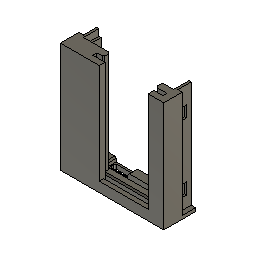
POWERDIAG_OBI_CASE_1 (Autodesk Fusion 360 design; units mm, degrees)
part number: 2026-08-31-19-42-01-999
Autodesk Fusion 360 part; units mm, degrees
note: some values were not read from the file. Set by a fixed rule: which sketch regions a step uses.
sketch "Sketch1" plane through (0, 0, 0) normal (0, 0, 1) x (1, 0, 0)
  line L0 (0, 0) -> (46.5, 0)
  line L1 (46.5, 0) -> (46.5, 14.3)
  line L2 (46.5, 14.3) -> (0, 14.3)
  line L3 (0, 14.3) -> (0, 0)
  line L4 (0, 2.6) -> (46.5, 2.6)
  line L5 (3, 14.3) -> (3, 0)
  line L6 (43.5, 14.3) -> (43.5, 0)
  line L7 (0, 4.4) -> (46.5, 4.4)
  line L8 (0, 7.4) -> (46.5, 7.4)
  line L9 (10.8, 10.6) -> (19.8, 10.6)
  line L10 (19.8, 10.6) -> (19.8, 14.3)
  line L11 (19.8, 14.3) -> (10.8, 14.3)
  line L12 (10.8, 14.3) -> (10.8, 10.6)
  line L13 (4, 10.6) -> (4, 9)
  line L14 (4, 9) -> (3, 9)
  line L15 (3, 9) -> (3, 11)
  line L16 (42.5, 10.6) -> (42.5, 9)
  line L17 (42.5, 9) -> (43.5, 9)
  line L18 (43.5, 9) -> (43.5, 11)
  line L19 (6.8, 14.3) -> (23.8, 14.3)
  line L20 (43.5, 10.6) -> (3, 10.6)
  line L21 (11.2, 13.45) -> (19.4, 13.45)
  line L22 (19.4, 13.45) -> (19.4, 10.95)
  line L23 (19.4, 10.95) -> (11.2, 10.95)
  line L24 (11.2, 10.95) -> (11.2, 13.45)
  line L25 (12, 4.4) -> (12, 2.6)
  line L26 (15, 7.4) -> (15, 4.4)
  line L27 (38.5, 7.4) -> (38.5, 4.4)
  line L28 (17.5, 2.6) -> (17.5, 0)
  line L29 (39.5, 2.6) -> (39.5, 0)
  line L30 (4, 10.6) -> (4, 14.3)
  line L31 (42.5, 10.6) -> (42.5, 14.3)
  dimension "d3" = 2.6
  dimension "d4" = 3
  dimension "d5" = 3
  dimension "d7" = 1.8
  dimension "d8" = 3
  dimension "d9" = 3.2
  dimension "d10" = 3.7
  dimension "d11" = 9
  dimension "d12" = 7.8
  dimension "d13" = 40.5
  dimension "d23" = 1
  dimension "d24" = 1.6
  dimension "d25" = 1.6
  dimension "d26" = 1
  dimension "d34" = 8.2
  dimension "d35" = 2.5
  dimension "d36" = 0.4
  dimension "d37" = 0.85
  dimension "d42" = 9
  dimension "d43" = 12
  dimension "d44" = 5
  dimension "d45" = 14.5
  dimension "d46" = 4
  constraint horizontal L0
  constraint vertical L1
  constraint horizontal L2
  constraint vertical L3
  constraint coincident L0.start L3.end
  constraint coincident L3 L4.start
  constraint coincident L1 L4.end
  constraint perpendicular L1 L4
  constraint coincident L2 L5.start
  constraint coincident L0 L5.end
  constraint perpendicular L0 L5
  constraint coincident L2 L6.start
  constraint coincident L0 L6.end
  constraint perpendicular L0 L6
  constraint coincident L1 L7.end
  constraint perpendicular L1 L7
  constraint coincident L3 L8.start
  constraint perpendicular L6 L8
  constraint coincident L1 L8.end
  constraint horizontal L9
  constraint vertical L10
  constraint horizontal L11
  constraint vertical L12
  constraint vertical L13
  constraint horizontal L14
  constraint vertical L15
  constraint coincident L5 L15.end
  constraint vertical L16
  constraint horizontal L17
  constraint vertical L18
  constraint coincident L6 L18.end
  constraint horizontal L19
  constraint horizontal L20
  constraint collinear L9 L20
  constraint horizontal L21
  constraint vertical L22
  constraint horizontal L23
  constraint vertical L24
  constraint coincident L7 L25.start
  constraint coincident L4 L25.end
  constraint perpendicular L7 L25
  constraint coincident L8 L26.start
  constraint coincident L7 L26.end
  constraint perpendicular L7 L26
  constraint coincident L8 L27.start
  constraint coincident L7 L27.end
  constraint perpendicular L7 L27
  constraint coincident L4 L28.start
  constraint coincident L0 L28.end
  constraint perpendicular L0 L28
  constraint coincident L4 L29.start
  constraint coincident L0 L29.end
  constraint perpendicular L0 L29
  constraint collinear L11 L19
  constraint collinear L2 L11
  constraint coincident L15 L20.end
  constraint coincident L16.start L20
  constraint coincident L13.start L20
  constraint coincident L2 L30.end
  constraint perpendicular L2 L30
  constraint coincident L2 L31.end
  constraint perpendicular L2 L31
  measures "d3" distance of L0 L4
  measures "d4" distance of L3 L5
  measures "d5" distance of L1 L6
  measures "d7" distance of L4 L7
  measures "d8" distance of L7 L8
  measures "d9" distance of L8 L9
  measures "d10" distance of L9.start L11.end
  measures "d11" distance of L10 L12
  measures "d12" distance of L5 L12
  measures "d13" distance of L5 L6
  measures "d23" distance of L5 L13
  measures "d24" distance of L8 L14
  measures "d25" distance of L8 L17
  measures "d26" distance of L16 L18
  measures "d34" distance of L22 L24
  measures "d35" distance of L21 L23
  measures "d36" distance of L12 L24
  measures "d37" distance of L11 L21
  measures "d42" distance of L5 L25
  measures "d43" distance of L5 L26
  measures "d44" distance of L6 L27
  measures "d45" distance of L5 L28
  measures "d46" distance of L6 L29
extrude "Extrude1" add sketch "Sketch1" against normal blind 2
extrude "Extrude2" add sketch "Sketch1" along normal blind 3 contours L0 L3 L4 L5 | L0 L4 L5 L28 | L3 L4 L5 L7 | L0 L4 L28 L29 | L3 L5 L7 L8 | L0 L4 L6 L29 | L5 L7 L8 L26 | L2 L3 L5 L8 L15 | L0 L1 L4 L6 | L1 L4 L6 L7 | L7 L8 L26 L27 | L6 L7 L8 L27 | L1 L6 L7 L8 | L1 L2 L6 L8 L18
sketch "Sketch2" plane through (0, 0, 3) normal (0, 0, 1) x (-1, 0, 0)
  line L0 (-3, -4.4) -> (-43.5, -4.4)
  line L1 (-43.5, -4.4) -> (-43.5, -2.6)
  line L2 (-43.5, -2.6) -> (-3, -2.6)
  line L3 (-3, -2.6) -> (-3, -4.4)
  line L4 (0, -14.3) -> (0, 0)
  line L5 (0, 0) -> (-46.5, 0)
  line L6 (-46.5, 0) -> (-46.5, -14.3)
  line L7 (-43.5, -14.3) -> (-43.5, -7.4)
  line L8 (-43.5, -7.4) -> (-3, -7.4)
  line L9 (-3, -7.4) -> (-3, -14.3)
  line L10 (-15, -7.4) -> (-15, -4.4)
  line L11 (-3, -14.3) -> (-3, 0)
  line L12 (-38.5, -7.4) -> (-38.5, -4.4)
  line L13 (-43.5, -14.3) -> (-43.5, 0)
  line L14 (-12, -4.4) -> (-12, -2.6)
  line L15 (-38.5, -7.4) -> (-38.5, -4.4)
  line L16 (-15, -7.4) -> (-15, -4.4)
  line L17 (-17.5, -2.6) -> (-17.5, 0)
  line L18 (-39.5, -2.6) -> (-39.5, 0)
  line L19 (-3, -14.3) -> (0, -14.3)
  line L20 (-46.5, -14.3) -> (-43.5, -14.3)
  dimension "d18" = 12
  dimension "d19" = 5
  constraint coincident L8 L10.start
  constraint coincident L0 L10.end
  constraint perpendicular L0 L10
  constraint coincident L8 L12.start
  constraint coincident L0 L12.end
  constraint perpendicular L0 L12
  measures "d18" distance of L10 L11
  measures "d19" distance of L12 L13
extrude "Extrude3" add sketch "Sketch2" along normal blind 45 contours L0 L8 L10 L11 L16 | L0 L2 L3 L11 L14 | L3 L4 L5 L9 L11 L19 | L2 L5 L11 L17 | L0 L8 L12 L13 L15 | L1 L5 L6 L7 L13 L20 | L2 L5 L13 L18
extrude "Extrude4" add sketch "Sketch1" along normal blind 45 contours L5 L13 L14 L15 L20 | L2 L5 L15 L20 L30 | L6 L16 L17 L18 L20 | L2 L6 L18 L20 L31
chamfer "Chamfer1" distance 0.6 angle 45 8 edges at (4, 9, 22.5) (15, 7.4, 25.5) (15, 4.4, 25.5) (42.5, 9, 22.5) (38.5, 7.4, 25.5) (38.5, 4.4, 25.5) (28.5, 2.6, 3) (26.75, 4.4, 3)
extrude "Extrude5" add sketch "Sketch1" along normal blind 2 contours L2 L5 L15 L20 L30 | L2 L12 L19 L20 L30 | L2 L6 L18 L20 L31 | L2 L10 L19 L20 L31
fillet "Fillet1" radius 0.8 4 edges at (11.2, 10.95, -1) (19.4, 10.95, -1) (19.4, 13.45, -1) (11.2, 13.45, -1)
extrude "Extrude6" cut sketch "Sketch1" against normal blind 0.5 contours L5 L6 L8 L9 L13 L14 L16 L17 L20
chamfer "Chamfer2" distance 0.6 angle 45 2 edges at (10.8, 12.45, 2) (19.8, 12.45, 2)
sketch "Sketch3" plane through (0, 0, 0) normal (-1, 0, 0) x (0, -1, 0)
  line L0 (-14.3, 48) -> (-14.3, -2)
  line L1 (-14.3, -2) -> (0, -2)
  line L2 (0, -2) -> (0, 48)
  line L3 (0, 48) -> (-14.3, 48)
  line L4 (-8.3, 0) -> (-14.3, 0)
  line L5 (-14.3, 0) -> (-14.3, 48)
  line L6 (-14.3, 48) -> (-8.3, 48)
  line L7 (-8.3, 48) -> (-8.3, 0)
  line L8 (-14.3, 0) -> (0, 0)
  dimension "d52" = 6
  constraint horizontal L4
  constraint vertical L5
  constraint horizontal L6
  constraint vertical L7
  constraint coincident L0.start L3.end
  constraint collinear L4 L8
  measures "d52" distance of L5 L7
extrude "Extrude7" cut sketch "Sketch3" against normal blind 2 contours L0 L3 L4 L5 L6 L7 L8
sketch "Sketch4" plane through (46.5, 0, 0) normal (1, 0, 0) x (0, 1, 0)
  line L0 (0, 48) -> (0, -2)
  line L1 (0, -2) -> (14.3, -2)
  line L2 (14.3, -2) -> (14.3, 48)
  line L3 (14.3, 48) -> (0, 48)
ref_plane "WorkPlane1" through (23.25, 7.15, 23) normal (-1, 0, 0) x (0, 1, 0)
mirror "Mirror1" about plane through (23.25, 7.15, 23) normal (-1, 0, 0) of "Extrude7"
sketch "Sketch5" plane through (2, 0, 0) normal (-1, 0, 0) x (0, -1, 0)
  line L0 (-14.3, 48) -> (-14.3, 0)
  line L1 (-14.3, 0) -> (-8.3, 0)
  line L2 (-8.3, 0) -> (-8.3, 48)
  line L3 (-8.3, 48) -> (-14.3, 48)
  line L4 (-10.3, 5) -> (-12.3, 5)
  line L5 (-12.3, 5) -> (-12.3, 10)
  line L6 (-12.3, 10) -> (-10.3, 10)
  line L7 (-10.3, 10) -> (-10.3, 5)
  dimension "d57" = 2
  dimension "d58" = 2
  dimension "d59" = 5
  dimension "d60" = 5
  constraint horizontal L4
  constraint vertical L5
  constraint horizontal L6
  constraint vertical L7
  measures "d57" distance of L4.start L4.end
  measures "d58" distance of L0 L5
  measures "d59" distance of L1 L4
  measures "d60" distance of L4 L6
extrude "Extrude8" cut sketch "Sketch5" against normal blind 1 contours L4 L5 L6 L7
pattern_linear "R-Pattern1" count 2 spacing 30 along (0, 0, 1) of "Extrude8"
mirror "Mirror2" about plane through (23.25, 7.15, 23) normal (-1, 0, 0) of "Extrude8", "R-Pattern1"
chamfer "Chamfer3" distance 0.5 angle 45 3 edges at (0, 7.15, -2) (23.25, 0, -2) (46.5, 7.15, -2)
